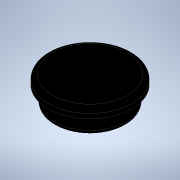
# Autodesk Inventor part: sensor_2
Saved by Autodesk Inventor 2021 (Build 250183000, 183)
## iProperties
Created: 2024-10-05
Part Number: sensor_2
Material: Generic
Document SubType Name: Modeling
Designer: hojan
Density: 1 g/cm^3
Appearance: Default
Author: hojan
Autodesk Inventor part; units mm, degrees
ref_plane "YZ Plane" through (0, 0, 0) normal (1, 0, 0) x (0, 1, 0)
ref_plane "XZ Plane" through (0, 0, 0) normal (0, 1, 0) x (-1, 0, 0)
ref_plane "XY Plane" through (0, 0, 0) normal (0, 0, 1) x (1, 0, 0)
sketch "Boceto1" plane through (0, 0, 0) normal (0, 1, 0) x (-1, 0, 0)
  circle A0 centre (0, 0) radius 4.5
  dimension "d0" = 9
  constraints: 1 centre point, 1 coincident
  measures "d0" diameter of A0
extrude "Extrusión1" add sketch "Boceto1" along normal blind 1
fillet "Empalme1" radius 0.5 1 edges at (4.5, 1, 0)
sketch "Boceto2" plane through (0, 0, 0) normal (0, -1, 0) x (1, 0, 0)
  circle A0 centre (0, 0) radius 3.9
  dimension "d4" = 7.8
  constraints: 1 centre point, 1 coincident
  measures "d4" diameter of A0
extrude "Extrusión2" add sketch "Boceto2" along normal blind 2
fillet "Empalme2" radius 0.5 1 edges at (-3.9, -2, 0)
